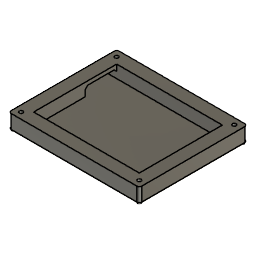
bottom (Autodesk Fusion 360 design; units mm, degrees)
part number: 2026-02-21-15-50-16-128
Autodesk Fusion 360 part; units mm, degrees
sketch "Schizzo1" plane through (0, 0, 0) normal (0, 0, 1) x (1, 0, 0)
  line L0 (0, 0) -> (84, 0)
  line L1 (84, 0) -> (84, 66)
  line L2 (84, 66) -> (0, 66)
  line L3 (0, 66) -> (0, 0)
  line L4 (-10, -10) -> (94, -10)
  line L5 (94, -10) -> (94, 76)
  line L6 (94, 76) -> (-10, 76)
  line L7 (-10, 76) -> (-10, -10)
  circle A0 centre (-5, 71) radius 1.45
  circle A1 centre (-5, -5) radius 1.45
  circle A2 centre (89, -5) radius 1.45
  circle A3 centre (88.5374, 71) radius 1.45
  line L8 (0, 66) -> (84, 66)
  line L9 (84, 66) -> (84, 0)
  line L10 (84, 0) -> (0, 0)
  line L11 (0, 0) -> (0, 66)
  dimension "d1" = 84
  dimension "d2" = 66
  dimension "d3" = 10
  dimension "d4" = 2.9
  dimension "d5" = 2.9
  dimension "d6" = 2.9
  dimension "d7" = 5
  dimension "d8" = 5
  dimension "d9" = 5
  dimension "d10" = 5
  dimension "d11" = 5
  dimension "d12" = 2.9
  dimension "d13" = 5
  dimension "d14" = 5.4626
  constraint horizontal L0
  constraint vertical L1
  constraint horizontal L2
  constraint vertical L3
  constraint coincident L0.start L3.end
  constraint horizontal L8
  constraint vertical L9
  constraint horizontal L10
  constraint vertical L11
  measures "d1" distance of L0.start L0.end
  measures "d2" distance of L0.start L2.end
  measures "d4" diameter of A0
  measures "d5" diameter of A1
  measures "d6" diameter of A2
  measures "d7" distance of L4 A2.centre
  measures "d8" distance of L5 A2.centre
  measures "d9" distance of L4 A1.centre
  measures "d10" distance of L6 A0.centre
  measures "d11" distance of L7 A0.centre
  measures "d12" diameter of A3
  measures "d13" distance of L6 A3.centre
  measures "d14" distance of L5 A3.centre
extrude "Estrusione1" add sketch "Schizzo1" along normal blind 13
sketch "Schizzo2" plane through (0, 0, 0) normal (0, 0, 1) x (1, 0, 0)
  line L0 (0, 0) -> (84, 0)
  line L1 (84, 0) -> (84, 66)
  line L2 (84, 66) -> (0, 66)
  line L3 (0, 66) -> (0, 0)
  constraint horizontal L0
  constraint vertical L1
  constraint horizontal L2
  constraint vertical L3
  constraint coincident L0.start L3.end
extrude "Estrusione2" add sketch "Schizzo2" along normal blind 3
sketch "Sketch3" plane through (-10, 0, 0) normal (-1, 0, 0) x (0, -1, 0)
  line L0 (-76, 0) -> (10, 0)
  line L1 (10, 0) -> (10, 13)
  line L2 (10, 13) -> (-76, 13)
  line L3 (-76, 13) -> (-76, 0)
  line L4 (-66, 3) -> (-41, 3)
  line L5 (-41, 3) -> (-41, 8)
  line L6 (-41, 8) -> (-43, 10)
  line L7 (-43, 10) -> (-64, 10)
  line L8 (-64, 10) -> (-66, 8)
  line L9 (-66, 8) -> (-66, 3)
  constraint horizontal L4
  constraint perpendicular L4 L5
  constraint perpendicular L5 L7
  constraint perpendicular L6 L8
  constraint perpendicular L4 L9
extrude "Extrude3" cut sketch "Sketch3" against normal blind 10 contours L4 L5 L6 L7 L8 L9
fillet "Fillet1" radius 2 4 edges at (94, 33, 0) (42, -10, 0) (-10, 33, 0) (42, 76, 0)
fillet "Fillet2" radius 2 8 edges at (-9.4142, -9.4142, 0.5858) (-10, -10, 7.5) (93.4142, -9.4142, 0.5858) (94, -10, 7.5) (93.4142, 75.4142, 0.5858) (94, 76, 7.5) (-9.4142, 75.4142, 0.5858) (-10, 76, 7.5)
